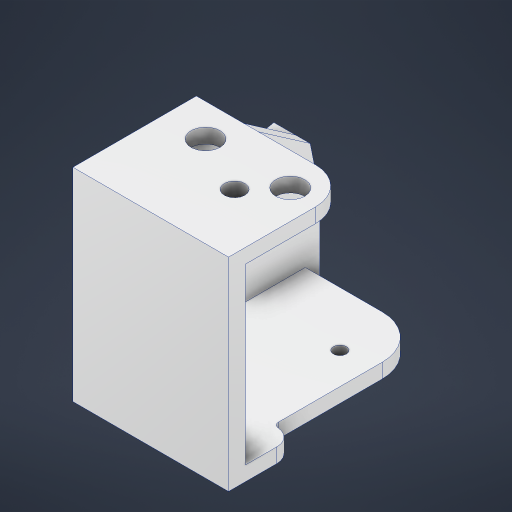
# Autodesk Inventor part: DC23[R][FD1]
Saved by Autodesk Inventor 2024 (Build 280153000, 153)
## iProperties
Created: 2022-10-25
Part Number: DC23[R][FD1]
Material: Aluminio 6061
Document SubType Name: Modeling
Designer: juanr
Density: 2.7 g/cm^3
Appearance: Aluminio - Plano
Mass: 248.976 g
Surface Area: 332.545 cm^2
Volume: 92.2132 cm^3
Author: juanr
Autodesk Inventor part; units mm, degrees
ref_plane "YZ Plane" through (0, 0, 0) normal (1, 0, 0) x (0, 1, 0)
ref_plane "XZ Plane" through (0, 0, 0) normal (0, 1, 0) x (-1, 0, 0)
ref_plane "XY Plane" through (0, 0, 0) normal (0, 0, 1) x (1, 0, 0)
sketch "Sketch1" plane through (0, 0, 0) normal (0, 1, 0) x (-1, 0, 0)
  line L0 (0, -25.5) -> (-34.15, -25.5)
  line L1 (-34.15, -25.5) -> (-34.15, 0)
  line L2 (-34.15, 0) -> (-34.15, 25.5)
  line L3 (-34.15, 25.5) -> (0, 25.5)
  line L4 (0, 25.5) -> (34.15, 25.5)
  line L5 (34.15, 25.5) -> (34.15, 0)
  line L6 (34.15, 0) -> (34.15, -25.5)
  line L7 (34.15, -25.5) -> (0, -25.5)
  point P0 (0, 0)
  constraints: 16 end point, 3 perpendicular, 2 point on line, 1 horizontal, 1 vertical
extrude "Extrusion1" add sketch "Sketch1" along normal blind 7
sketch "Sketch3" plane through (-34.15, 0, 25.5) normal (0, 0, 1) x (1, 0, 0)
  line L0 (0, 0) -> (0, -78.85)
  point P0 (34.15, 0)
  dimension "d7" = 78.85
  constraints: 2 end point, 1 vertical
  measures "d7" distance of L0.start L0.end
sketch "Sketch4" plane through (-34.15, 0, -25.5) normal (-1, 0, 0) x (0, 0, 1)
  line L0 (51, 0) -> (51, -78.85)
  line L1 (51, -78.85) -> (-39, -78.85)
  line L2 (-39, -78.85) -> (-39, -71.85)
  line L3 (0, 0) -> (-39, -71.85)
  line L4 (0, 0) -> (51, 0)
  point P0 (25.5, 0)
  dimension "d10" = 90
  dimension "d11" = 7
  constraints: 10 end point, 2 horizontal, 2 vertical
  measures "d10" distance of L0.end L1.end
  measures "d11" distance of L1.end L2.end
extrude "Extrusion2" add sketch "Sketch4" against normal blind 7
sketch "Sketch6" plane through (0, 7, 0) normal (0, 1, 0) x (1, 0, 0)
  line L0 (34.15, -25.5) -> (34.15, 25.5) projected
  line L1 (34.15, 25.5) -> (34.15, 0)
  line L2 (-34.15, 25.5) -> (-34.15, -25.5) projected
  circle A0 centre (8.15, 0) radius 5
  point P0 (0, 0)
  dimension "d20" = 10
  constraints: 2 end point, 1 centre point, 1 midpoint
  measures "d20" diameter of A0
extrude "Extrusion4" cut sketch "Sketch6" against normal blind 10
sketch "Sketch7" plane through (-27.15, 0, -25.5) normal (1, 0, 0) x (0, 0, -1)
  line L0 (-51, -78.85) -> (39, -78.85) projected
  line L1 (-51, -78.85) -> (39, -78.85)
  line L2 (39, -78.85) -> (39, -71.85) projected
  line L3 (39, -78.85) -> (39, -71.85)
  line L4 (39, -71.85) -> (-51, -71.85)
  line L5 (-51, 0) -> (-51, -78.85) projected
  line L6 (-51, -78.85) -> (-51, -71.85)
  point P0 (-25.5, 0)
  constraints: 8 end point, 2 perpendicular, 1 collinear, 1 horizontal, 1 point on line
sketch "Sketch8" plane through (0, 0, 0) normal (0, -1, 0) x (1, 0, 0)
  circle A0 centre (8.15, 0) radius 5 projected
  line L0 (8.15, 18.5) -> (34.15, 18.5)
  line L1 (34.15, 25.5) -> (34.15, -25.5) projected
  line L2 (8.15, 25.5) -> (34.15, 25.5)
  line L3 (8.15, 25.5) -> (-27.15, 25.5)
  line L4 (-27.15, 25.5) -> (-27.15, -25.5) projected
  line L5 (8.15, 18.5) -> (-27.15, 18.5)
  line L6 (34.15, 25.5) -> (34.15, 18.5)
  line L7 (-27.15, 25.5) -> (-27.15, 18.5)
  point P0 (0, 0)
  constraints: 12 end point, 2 collinear, 2 point on line, 1 horizontal, 1 parallel
extrude "Extrusion6" add sketch "Sketch7" along normal blind 58.5
extrude "Extrusion7" add sketch "Sketch8" along normal blind 78.75 contours L5 L4 L3 L2 L1 L0
sketch "Sketch9" plane through (31.35, 0, -25.5) normal (1, 0, 0) x (0, 0, -1)
  line L0 (-51, -78.75) -> (-51, 7) projected
  line L1 (-44, 0) -> (-44, -71.85) projected
  line L2 (-51, -78.75) -> (-44, -78.75)
  line L3 (-44, -78.75) -> (-44, -71.85)
  line L4 (-44, -71.85) -> (-51, -71.85)
  line L5 (-51, -71.85) -> (-51, -78.75)
  point P0 (-25.5, 0)
  constraints: 8 end point, 2 parallel, 1 horizontal, 1 perpendicular
extrude "Extrusion8" cut sketch "Sketch9" along normal blind 10
sketch "Boceto11" plane through (-34.15, -78.85, -64.5) normal (0, -1, 0) x (1, 0, 0)
  line L0 (72.0718, 89.9914) -> (72.0718, 37.9883)
  line L1 (72.0718, 37.9883) -> (65.5278, 37.9883)
  line L2 (65.5278, 37.9883) -> (65.5278, 89.9914)
  line L3 (72.0718, 89.9914) -> (72.0718, 92.1751)
  line L4 (72.0718, 92.1751) -> (65.5278, 92.1751)
  line L5 (65.5278, 92.1751) -> (65.5278, 89.9914)
  point P0 (34.15, 64.5)
  constraints: 12 end point, 2 perpendicular, 1 parallel, 1 vertical
extrude "Extrusión9" cut sketch "Boceto11" against normal blind 1000
sketch "Boceto24" plane through (-27.15, 0, -25.5) normal (0, 0, -1) x (-1, 0, 0)
  line L0 (7, -71.85) -> (7, -78.85) projected
  line L1 (7, -78.35) -> (7, -78.85)
  line L2 (7, -78.85) -> (-58.5, -78.85) projected
  line L3 (-58.5, -78.85) -> (-58.5, -77.85)
  line L4 (-58.5, -71.85) -> (-58.5, -78.85) projected
  line L5 (-58.5, -77.85) -> (6, -77.85)
  line L6 (7, -77.85) -> (7, -78.85)
  line L7 (7, -78.85) -> (-58.8392, -78.85)
  line L8 (-58.5278, 7) -> (7, 7) projected
  line L9 (7, -78.85) -> (7, 7)
  line L10 (7, 7) -> (6, 7)
  line L11 (6, 6) -> (6, -77.85)
  line L12 (-58.5278, -71.85) -> (-58.5278, 7) projected
  line L13 (-58.5278, 7) -> (-58.5278, 6)
  line L14 (-58.5278, 6) -> (6, 6)
  line L15 (7, 0) -> (7, 7) projected
  line L16 (7, 6) -> (7, 7)
  line L17 (7, 7) -> (-58.5278, 7)
  point P0 (-27.15, 0)
  dimension "d65" = 1
  dimension "d66" = 1
  dimension "d67" = 1
  constraints: 24 end point, 7 perpendicular, 5 point on line, 1 collinear, 1 horizontal, 1 vertical
  measures "d65" distance of L2.end L3.end
  measures "d66" distance of L8.end L10.end
  measures "d67" distance of L8.start L13.end
extrude "Extrusión19" cut sketch "Boceto24" along normal mid plane 1000
sketch "Boceto27" plane through (31.3778, 0, -25.5) normal (0, 0, -1) x (-1, 0, 0)
  line L0 (0, -71.85) -> (0, 6) projected
  line L1 (0, 6) -> (0.228, 6)
  line L2 (0, 6) -> (64.5278, 6) projected
  line L3 (0.228, 6) -> (0.228, -77.85)
  line L4 (0.0278, -77.85) -> (64.5278, -77.85) projected
  line L5 (0.0278, -71.85) -> (0.0278, -77.85) projected
  line L6 (0.228, -77.85) -> (0.0278, -77.85)
  line L7 (0.0278, -77.85) -> (0, 6)
  line L8 (0, 6) -> (0, -77.85)
  line L9 (0, -77.85) -> (0.0278, -77.85)
  point P0 (31.3778, 0)
  dimension "d73" = 0.228
  constraints: 12 end point, 3 perpendicular, 3 point on line, 1 horizontal
  measures "d73" distance of L0.end L1.end
extrude "Extrusión21" cut sketch "Boceto27" along normal mid plane 1000
sketch "Boceto31" plane through (-33.15, 0, -25.5) normal (-1, 0, 0) x (0, 0, 1)
  circle A0 centre (64.38, -38.5153) radius 2.6
  point P0 (25.5, 0)
  point P1 (64.38, -49.4573)
  constraints: 1 centre point
sketch "Boceto32" plane through (-27.15, -71.85, 18.5) normal (0, 1, 0) x (1, 0, 0)
  circle A0 centre (47, 71.5) radius 5 projected
  circle A1 centre (47, 71.5) radius 5
  line L0 (52, 71.5) -> (58.2998, 71.5)
  line L1 (67, 83) -> (67, -7)
  line L2 (58.2998, -7) -> (-6, -7) projected
  line L3 (67, -7) -> (58.2998, -7)
  line L4 (58.2998, -7) -> (58.2998, 83)
  line L5 (47, 76.5) -> (47, 83)
  line L6 (-6, 83) -> (0, 83) projected
  line L7 (-6, 83) -> (-6, 91.5)
  line L8 (-6, 91.5) -> (67, 91.5)
  line L9 (67, 91.5) -> (67, 83)
  line L10 (-6, 83) -> (58.2998, 83)
  point P0 (27.15, 18.5)
  constraints: 18 end point, 2 perpendicular, 2 point on circle, 2 point on line, 2 vertical, 1 centre point, 1 coincident, 1 collinear, 1 horizontal
extrude "Extrusión23" add sketch "Boceto32" against normal blind 6 contours L4 L10 L6 L7 L8 L9 L1 L3
sketch "Boceto33" plane through (-33.15, -77.85, 25.5) normal (-1, 0, 0) x (0, 0, 1)
  line L0 (0, 83.85) -> (0, 0) projected
  line L1 (0, 74.4354) -> (10.1255, 74.4354)
  line L2 (10.1255, 74.4354) -> (10.1255, 56.6115)
  line L3 (10.9445, 54.9975) -> (18.0243, 49.8171)
  line L4 (18.8039, 48.5979) -> (20.1084, 42.1205)
  line L5 (0, 11.6181) -> (18.1478, 11.6181)
  line L6 (20.1478, 13.6181) -> (20.1478, 41.7256)
  arc A0 (10.1255, 56.6115) -> (10.9445, 54.9975) centre (12.1255, 56.6115) ccw
  arc A1 (18.8039, 48.5979) -> (18.0243, 49.8171) centre (16.8433, 48.203) ccw
  arc A2 (20.1478, 41.7256) -> (20.1084, 42.1205) centre (18.1478, 41.7256) ccw
  arc A3 (18.1478, 11.6181) -> (20.1478, 13.6181) centre (18.1478, 13.6181) ccw
  point P0 (-25.5, 77.85)
  dimension "d91" = 2
  constraints: 12 end point, 8 point on circle, 8 tangent, 4 centre point, 3 equal radius, 2 horizontal, 2 perpendicular, 2 point on line
  measures "d91" radius of A0
extrude "Extrusión24" add sketch "Boceto33" against normal blind 6
extrude "Extrusión25" cut sketch "Boceto31" against normal blind 6
sketch "Boceto34" plane through (-27.15, -77.85, 25.5) normal (1, 0, 0) x (0, 0, -1)
  line L0 (-18.1478, 11.6181) -> (-21.8775, 11.6181)
  line L1 (-21.8775, 11.6181) -> (-21.8775, 48.067)
  line L2 (-21.8775, 48.067) -> (-10.1255, 56.8358)
  line L3 (-10.1255, 74.4354) -> (-10.1255, 56.6115) projected
  line L4 (-10.1255, 56.8358) -> (-10.1255, 48.9642)
  line L5 (-10.1255, 48.9642) -> (-16.6729, 42.1735)
  line L6 (-16.6729, 42.1735) -> (-18.1478, 11.6181)
  point P0 (25.5, 77.85)
  constraints: 12 end point, 1 horizontal, 1 perpendicular, 1 point on line, 1 vertical
extrude "Extrusión26" add sketch "Boceto34" against normal blind 6
fillet "Empalme5" radius 10 3 edges at (-30.15, -21.0142, 35.6255) (-30.15, -29.783, 47.3775) (-30.15, -66.2319, 47.3775)
sketch "Boceto37" plane through (-33.15, 6, 25.5) normal (0, 1, 0) x (1, 0, 0)
  circle A0 centre (52.2998, 37.5) radius 6
  circle A1 centre (17.3, 37.5) radius 6
  line L0 (64.2998, 37.5) -> (52.2998, 37.5)
  circle A2 centre (52.2998, 37.5) radius 6
  dimension "d109" = 12
  dimension "d110" = 12
  dimension "d229" = 12
  constraints: 3 centre point, 2 end point, 1 coincident
  measures "d109" diameter of A0
  measures "d110" diameter of A1
  measures "d229" diameter of A2
extrude "Extrusión29" cut sketch "Boceto37" against normal blind 6.5
sketch "Boceto39" plane through (-27.15, -71.85, 18.5) normal (0, 1, 0) x (1, 0, 0)
  line L0 (58.2998, -7) -> (58.2998, 0)
  line L1 (58.2998, 44) -> (58.2998, 91.5)
  line L2 (-6, 91.5) -> (67, 91.5) projected
  line L3 (0, 0) -> (58.2998, 0) projected
  line L4 (58.2998, 0) -> (58.2998, -7) projected
  line L5 (58.2998, -7) -> (67, -7) projected
  line L6 (58.2998, -7) -> (67, -7)
  line L7 (67, 91.5) -> (-6, 91.5) projected
  line L8 (67, -7) -> (67, 91.5)
  line L9 (67, 91.5) -> (58.2998, 91.5)
  line L10 (58.2998, 0) -> (58.2998, 44)
  point P0 (27.15, 18.5)
  constraints: 12 end point, 3 collinear, 2 point on line, 1 perpendicular, 1 vertical
extrude "Extrusión31" cut sketch "Boceto39" against normal blind 10
sketch "Boceto41" plane through (-27.15, -71.85, 18.5) normal (0, 1, 0) x (1, 0, 0)
  circle A0 centre (36.8, 60.5) radius 2.7
  line L0 (-6, -7) -> (-6, 44) projected
  line L1 (-6, -7) -> (36.8, -7)
  line L2 (36.8, -7) -> (36.8, 60.5)
  line L3 (36.8, 60.5) -> (-6, 60.5)
  line L4 (-6, 60.5) -> (-6, -7)
  point P0 (27.15, 18.5)
  point P1 (58.2998, 91.5)
  dimension "d126" = 5.4
  dimension "d213" = 42.8
  dimension "d214" = 67.5
  constraints: 8 end point, 2 parallel, 1 centre point, 1 horizontal, 1 perpendicular
  measures "d126" diameter of A0
  measures "d213" distance of L3.end L2.end
  measures "d214" distance of L2.end L1.end
extrude "Extrusión32" cut sketch "Boceto41" against normal blind 10 contours A0 L2 L3 | L3 L2 A0
sketch "Sketch42" plane through (-27.15, -71.85, 18.5) normal (0, 1, 0) x (1, 0, 0)
  circle A0 centre (36.8, 60.5) radius 2.7 projected
  line L0 (36.8, 63.2) -> (36.8, 60.5)
  circle A1 centre (31.7998, 65) radius 18
  line L1 (0, 0) -> (0, 83) projected
  line L2 (0, 83) -> (31.7998, 83)
  line L3 (58.2998, 91.5) -> (-6, 91.5) projected
  line L4 (49.7998, 65) -> (49.7998, 0)
  line L5 (58.2998, 0) -> (0, 0) projected
  line L6 (0, 0) -> (58.2998, 0) projected
  line L7 (49.7998, 0) -> (58.2998, 0)
  line L8 (58.2998, 91.5) -> (58.2998, -7) projected
  line L9 (58.2998, 0) -> (58.2998, 91.5)
  line L10 (0, 83) -> (0, 44) projected
  line L11 (0, 83) -> (-6, 83)
  line L12 (-6, 91.5) -> (-6, 83) projected
  line L13 (-6, 83) -> (-6, 91.5)
  line L14 (58.2998, 91.5) -> (58.2998, 0) projected
  line L15 (-6, 91.5) -> (58.2998, 91.5)
  point P0 (27.15, 18.5)
  point P1 (58.2998, -7)
  dimension "d129" = 36
  constraints: 16 end point, 3 vertical, 2 collinear, 2 point on circle, 1 centre point, 1 horizontal, 1 parallel, 1 perpendicular, 1 point on line, 1 vertical alignment, 3 other
  measures "d129" diameter of A1
extrude "Extrusion33" cut sketch "Sketch42" against normal blind 10 contours A1 L2 L11 L12 L3 L8 L5 L4
sketch "Sketch43" plane through (-27.15, -71.85, 18.5) normal (0, 0, -1) x (-1, 0, 0)
  line L0 (6, -6) -> (-58.2998, -6) projected
  line L1 (0, 0) -> (-49.7998, 0) projected
  line L2 (-58.2998, -6) -> (-49.7998, -6)
  line L3 (-49.7998, -6) -> (-49.7998, 0)
  line L4 (-49.7998, 0) -> (-58.2998, 0)
  line L5 (-58.2998, 0) -> (-58.2998, -6)
  point P0 (-27.15, 71.85)
  constraints: 8 end point, 2 parallel, 1 horizontal, 1 perpendicular
extrude "Extrusion34" add sketch "Sketch43" along normal blind 20
fillet "Fillet7" radius 7 1 edges at (31.1498, -74.85, -1.5)
fillet "Fillet8" radius 2 1 edges at (22.6498, -74.85, -1.5)
sketch "Sketch44" plane through (-33.15, 0, -25.5) normal (-1, 0, 0) x (0, 0, 1)
  line L0 (68.8577, -26.7837) -> (65.1452, -24.0136) projected
  line L1 (61.1255, -3.4146) -> (51, -3.4146) projected
  line L2 (65.1452, -24.0136) -> (51, -24.0136)
  line L3 (51, -24.0136) -> (51, -3.4146)
  line L4 (51, -3.4146) -> (65.1452, -3.4146)
  line L5 (65.1452, -3.4146) -> (65.1452, -24.0136)
  point P0 (25.5, 0)
  constraints: 8 end point, 2 parallel, 1 horizontal, 1 perpendicular
extrude "Extrusion35" cut sketch "Sketch44" against normal blind 20
sketch "Sketch45" plane through (-33.15, 6, 25.5) normal (0, 1, 0) x (1, 0, 0)
  circle A0 centre (41.3, 25.5) radius 5 projected
  circle A1 centre (41.3, 25.5) radius 4.25
  circle A2 centre (41.3, 25.5) radius 5
  point P0 (33.15, 25.5)
  dimension "d138" = 8.5
  constraints: 2 centre point, 2 coincident, 1 concentric
  measures "d138" diameter of A1
extrude "Extrusion36" add sketch "Sketch45" against normal blind 6
sketch "Sketch47" plane through (-33.15, 0, -25.5) normal (-1, 0, 0) x (0, 0, 1)
  line L0 (-44.1201, -43.7798) -> (-41.0263, -28.4947)
  line L1 (-39, -71.85) -> (0, 0) projected
  line L2 (-41.0263, -28.4947) -> (0, 0)
  line L3 (0, 0) -> (-39, -71.85)
  line L4 (-44.1201, -43.7798) -> (-44.1201, -71.85)
  line L5 (-44.1201, -71.85) -> (-39, -71.85)
  point P0 (25.5, 0)
  constraints: 10 end point, 1 collinear, 1 perpendicular, 1 vertical
extrude "Extrusion37" add sketch "Sketch47" against normal blind 6
sketch "Sketch50" plane through (-33.15, 6, -25.5) normal (-1, 0, 0) x (0, 0, 1)
  line L0 (-44.1201, -49.7798) -> (-41.0263, -34.4947) projected
  line L1 (-41.0263, -34.4947) -> (-46.4891, -61.4839)
  line L2 (-39, -83.85) -> (51, -83.85) projected
  line L3 (-39, -83.85) -> (-46.4891, -83.85)
  line L4 (-46.4891, -83.85) -> (-46.4891, -61.4839)
  line L5 (-41.0263, -34.4947) -> (-39, -69.2782)
  line L6 (-39, -69.2782) -> (-39, -83.85)
  point P0 (25.5, -6)
  constraints: 10 end point, 1 collinear, 1 horizontal, 1 perpendicular, 1 vertical
extrude "Extrusion38" add sketch "Sketch50" against normal blind 6
sketch "Sketch51" plane through (-33.15, 6, -25.5) normal (-1, 0, 0) x (0, 0, 1)
  line L0 (-41.0263, -34.4947) -> (-46.4891, -61.4839) projected
  line L1 (-41.0263, -34.4947) -> (-46.4891, -61.4839)
  line L2 (-46.4891, -61.4839) -> (-15.8808, -61.4839)
  line L3 (-41.0263, -34.4947) -> (-15.8808, -34.4947)
  line L4 (-15.8808, -34.4947) -> (-15.8808, -61.4839)
  point P0 (25.5, -6)
  constraints: 8 end point, 2 horizontal, 1 collinear, 1 perpendicular
extrude "Extrusion39" add sketch "Sketch51" along normal blind 9
sketch "Sketch54" plane through (-33.15, 6, -25.5) normal (-1, 0, 0) x (0, 0, 1)
  line L0 (51, -72.2319) -> (51, -83.85) projected
  line L1 (51, -83.85) -> (86.3988, -83.85)
  line L2 (86.3988, -83.85) -> (86.3988, -18.2813)
  line L3 (86.3988, -18.2813) -> (51, -18.2813)
  line L4 (51, -18.2813) -> (51, -83.85)
  point P0 (25.5, -6)
  constraints: 8 end point, 2 parallel, 1 horizontal, 1 perpendicular
extrude "Extrusion41" cut sketch "Sketch54" against normal blind 26.989
sketch "Sketch55" plane through (-33.15, -55.4839, -71.9891) normal (0, 0.198384, -0.9801244) x (-1, 0, 0)
  line L0 (9, 6.0722) -> (9, 32.525) projected
  line L1 (9, 17.5562) -> (3.5, 17.5562)
  line L2 (9, 17.5562) -> (14.5, 17.5562) construction
  circle A0 centre (3.5, 17.5562) radius 2.55
  point P0 (-33.15, 68.6627)
  point P1 (9, 32.5248)
  dimension "d153" = 5.5
  dimension "d154" = 180
  dimension "d155" = 5.1
  constraints: 4 end point, 1 centre point, 1 coincident, 1 collinear, 1 horizontal, 1 perpendicular, 1 point on line
  measures "d153" distance of L1.start L1.end
  measures "d154" angle of L1 L2
  measures "d155" diameter of A0
extrude "Extrusion42" cut sketch "Sketch55" against normal blind 20
sketch "Sketch71" plane through (-33.15, -55.4839, -71.9891) normal (0, 0.198384, -0.9801244) x (-1, 0, 0)
  circle A0 centre (3.5, 17.5562) radius 2.55 projected
  line L0 (3.5, 17.5562) -> (3.5, 7.5762)
  line L1 (0, 27.5365) -> (9, 27.5365) projected
  line L2 (0, 79.6022) -> (0, -2.5812) projected
  line L3 (9, 27.5365) -> (9, 0) projected
  line L4 (0, 17.5562) -> (9, 17.5562)
  line L5 (9, 17.5562) -> (9, 7.5762)
  line L6 (9, 7.5762) -> (0, 7.5762)
  line L7 (0, 7.5762) -> (0, 17.5562)
  line L8 (9, 0) -> (0, 0)
  line L9 (0, 0) -> (0, 7.5762)
  line L10 (0, 7.5762) -> (9, 7.5762)
  line L11 (9, 7.5762) -> (9, 0)
  point P0 (-33.15, 68.6627)
  point P1 (0, 0)
  point P2 (0, 7.5762)
  dimension "d215" = 9.98
  constraints: 18 end point, 4 parallel, 3 perpendicular, 2 horizontal, 2 point on line
  measures "d215" distance of L0.start L0.end
extrude "Extrusion57" cut sketch "Sketch71" against normal blind 60 contours L6 L3 L8 L2
sketch "Sketch73" plane through (-42.15, 6, -25.5) normal (-1, 0, 0) x (0, 0, 1)
  line L0 (-46.4891, -61.4839) -> (-41.0263, -34.4947) projected
  line L1 (-41.0263, -34.4947) -> (-42.9731, -44.113)
  line L2 (-42.9731, -44.113) -> (-23.3706, -48.0807)
  line L3 (-41.0263, -34.4947) -> (-15.8808, -34.4947) projected
  line L4 (-20.6207, -34.4947) -> (-25.3836, -58.026)
  line L5 (-44.9861, -54.0583) -> (-15.8808, -59.9494) projected
  line L6 (-25.3836, -58.026) -> (-15.8808, -59.9494)
  line L7 (-20.6207, -34.4947) -> (-5.4041, -34.4947)
  line L8 (-5.4041, -34.4947) -> (-5.4041, -64.759)
  line L9 (-5.4041, -64.759) -> (-28.8644, -65.7075)
  line L10 (-28.8644, -65.7075) -> (-25.3836, -58.026)
  point P0 (25.5, -6)
  dimension "d218" = 20
  constraints: 16 end point, 3 perpendicular, 3 point on line, 1 horizontal
  measures "d218" distance of L1.end L2.end
sketch "Sketch74" plane through (-27.15, -55.4839, -71.9891) normal (0, 0.198384, -0.9801244) x (-1, 0, 0)
  line L0 (6, 27.5365) -> (0, 27.5365) projected
  line L1 (6, 27.5365) -> (16.0486, 27.5365)
  line L2 (16.0486, 27.5365) -> (16.0486, 36.432)
  line L3 (16.0486, 36.432) -> (6, 36.432)
  line L4 (6, 36.432) -> (6, 27.5365)
  point P0 (-27.15, 68.6627)
  constraints: 8 end point, 2 parallel, 1 horizontal, 1 perpendicular
extrude "Extrusion58" cut sketch "Sketch74" against normal blind 60
extrude "Extrusion59" cut sketch "Sketch73" against normal blind 9 contours L4 L3 L7 L8 L9 L10
fillet "Fillet10" radius 15 1 edges at (31.1498, 3, -25.5)
sketch "Sketch76" plane through (-33.15, -77.85, 25.5) normal (-1, 0, 0) x (0, 0, 1)
  line L0 (-95.9861, 29.7917) -> (-76.3836, 25.824) projected
  line L1 (-95.9861, 29.7917) -> (-95.9861, 0)
  line L2 (-97.4891, 0) -> (0, 0) projected
  line L3 (-97.4891, 22.3661) -> (-95.9861, 29.7917) projected
  line L4 (-97.4891, 0) -> (-97.4891, 22.3661)
  line L5 (-97.4891, 22.3661) -> (-95.9861, 29.7917)
  point P0 (-25.5, 77.85)
  constraints: 6 end point, 2 vertical, 1 collinear, 1 point on line
extrude "Extrusion60" cut sketch "Sketch76" against normal blind 9
body "Solid1"
